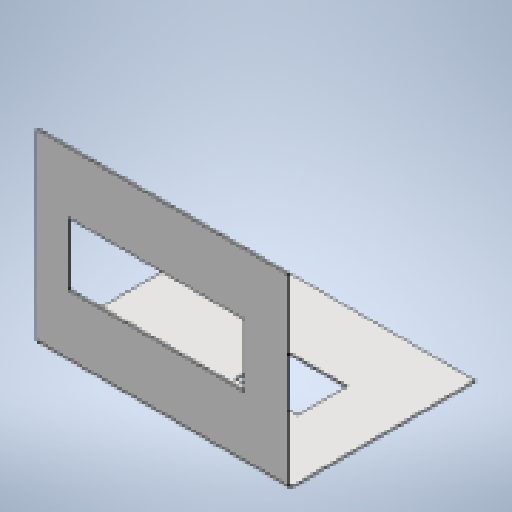
# Autodesk Inventor part: TKS 3004 BOTTOM DS box wall 1
Saved by Autodesk Inventor 2025 (Build 290162010, 162A)
## iProperties
Created: 2024-12-09
Part Number: TKS 3004 BOTTOM DS box wall 1
Material: Stainless Steel
Document SubType Name: Sheet Metal
Designer: user
Mass: 3269.02 g
Surface Area: 1007.63 cm^2
Volume: 408.627 cm^3
Density: 8 g/cm^3
Flat Pattern Width: 59.3927 cm
Flat Pattern Length: 40 cm
Flat Pattern Area: 2375.71 cm^2
Sheet Metal Rule: AISI304 3mm Die 32
Sheet Metal Width: 593,927 mm
Sheet Metal Length: 400,000 mm
Sheet Metal Area: 237570,973 mm^2
Appearance: Default
Author: user
Autodesk Inventor part; units mm, degrees
ref_plane "YZ Plane" through (0, 0, 0) normal (1, 0, 0) x (0, 1, 0)
ref_plane "XZ Plane" through (0, 0, 0) normal (0, 1, 0) x (-1, 0, 0)
ref_plane "XY Plane" through (0, 0, 0) normal (0, 0, 1) x (1, 0, 0)
sketch "Sketch1" plane through (0, 0, 0) normal (0, 0, 1) x (1, 0, 0)
  line L0 (200, 150) -> (-200, 150)
  line L1 (-200, 150) -> (-200, -150)
  line L2 (-200, -150) -> (200, -150)
  line L3 (200, -150) -> (200, 150)
  line L4 (200, 150) -> (-200, -150) construction
  line L5 (-200, 150) -> (200, -150) construction
  line L6 (106.4609, 40) -> (6.4609, 40)
  line L7 (6.4609, 40) -> (6.4609, -40)
  line L8 (6.4609, -40) -> (106.4609, -40)
  line L9 (106.4609, -40) -> (106.4609, 40)
  line L10 (106.4609, 40) -> (6.4609, -40) construction
  line L11 (6.4609, 40) -> (106.4609, -40) construction
  point P0 (0, 0)
  point P1 (0, 0)
  point P2 (56.4609, 0)
  point P3 (106.4609, 0)
  point P4 (200, 0)
  dimension "d32" = 300
  dimension "d33" = 400
  dimension "d34" = 100
  dimension "d35" = 80
  measures "d32" distance of L2.end L0.start
  measures "d33" distance of L1.end L2.end
  measures "d34" distance of L7.end L8.end
  measures "d35" distance of L8.end L6.start
extrude "Plate1" add sketch "Sketch1" along normal blind 3
sketch "Sketch6" plane through (200, -147, 0) normal (0, -1, 0) x (1, 0, 0)
  line L0 (-400, 0) -> (0, 0)
  line L1 (0, 0) -> (0, 300)
  line L2 (0, 300) -> (-400, 300)
  line L3 (-400, 300) -> (-400, 0)
  constraints: 6 end point, 1 horizontal, 1 perpendicular, 1 vertical
edge flange "Flange2" height 300 angle 90 thickness 3 bend radius 5 thickness toward (0, -1, 0) relief round relief width 3 relief depth 1.5 edges at (0, -150, 3) wall of the first edge with corners at (-200, -147, 0) (200, -147, 0) (200, -147, 300) (-200, -147, 300)
bend "Bend2"
corner "Corner2"
sketch "Sketch7" plane through (-200, -147, 300) normal (0, 1, 0) x (1, 0, 0)
  line L0 (0, 292) -> (400, 292) construction
  line L1 (400, 0) -> (400, 292) projected
  line L2 (0, 0) -> (400, 0) construction
  line L3 (0, 292) -> (0, 0) construction
  line L4 (50.3611, 97) -> (330.3611, 97)
  line L5 (330.3611, 97) -> (330.3611, 197)
  line L6 (330.3611, 197) -> (50.3611, 197)
  line L7 (50.3611, 197) -> (50.3611, 97)
  line L8 (50.3611, 97) -> (330.3611, 197) construction
  line L9 (330.3611, 97) -> (50.3611, 197) construction
  line L10 (400, 146) -> (0, 146) construction
  point P0 (200, 300)
  point P1 (190.3611, 147)
  dimension "d46" = 280
  dimension "d47" = 100
  dimension "d48" = 1
  constraints: 14 end point, 4 midpoint, 2 parallel, 1 horizontal, 1 perpendicular
  measures "d46" distance of L6.end L5.end
  measures "d47" distance of L5.end L4.end
  measures "d48" distance from line of L10 point (190.361, 147)
extrude "Cut2" cut sketch "Sketch7" against normal blind 3
equation "\"d49\" = Thickness"
equation "\"d2\" = Thickness"
equation "\"d36\" = BendReliefWidth"
equation "\"d37\" = BendReliefDepth"
equation "\"d38\" = MinimumRemnant"
equation "\"d39\" = TransitionRadius"
equation "\"d42\" = BendRadius"
equation "\"d43\" = CornerReliefSize"
equation "\"d44\" = GapSize"
equation "\"d45\" = JacobiRadiusSize"
equation "\"BendReliefWidth\" = Thickness"
equation "\"BendReliefDepth\" = 0.5 * Thickness"
equation "\"CornerReliefSize\" = 4 * Thickness"
equation "\"MinimumRemnant\" = 2 * Thickness"
equation "\"TransitionRadius\" = BendRadius"
equation "\"JacobiRadiusSize\" = BendRadius"
equation "\"GapSize\" = Thickness"
equation "\"Thickness\" = 3"
equation "\"BendRadius\" = 5"
body "Solid1"
